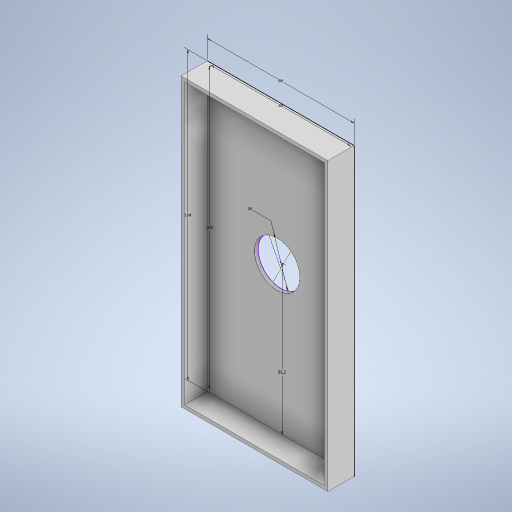
# Autodesk Inventor part: smartphone-holder-aperture26mm
Saved by Autodesk Inventor 2023 (Build 270158000, 158)
## iProperties
Created: 2023-10-02
Part Number: smartphone-holder-aperture26mm
Material: Generic
Document SubType Name: Modeling
Designer: nvladi
Density: 1 g/cm^3
Appearance: Default
Author: nvladi
Autodesk Inventor part; units mm, degrees
ref_plane "YZ Plane" through (0, 0, 0) normal (1, 0, 0) x (0, 1, 0)
ref_plane "XZ Plane" through (0, 0, 0) normal (0, 1, 0) x (-1, 0, 0)
ref_plane "XY Plane" through (0, 0, 0) normal (0, 0, 1) x (1, 0, 0)
sketch "Sketch1" plane through (0, 0, 0) normal (0, 0, 1) x (1, 0, 0)
  line L0 (40, -80) -> (-40, -80)
  line L1 (-40, -80) -> (-40, 80)
  line L2 (-40, 80) -> (40, 80)
  line L3 (40, 80) -> (40, -80)
  line L4 (40, -80) -> (-40, 80) construction
  line L5 (-40, -80) -> (40, 80) construction
  line L6 (42, -82) -> (-42, -82)
  line L7 (-42, -82) -> (-42, 82)
  line L8 (-42, 82) -> (42, 82)
  line L9 (42, 82) -> (42, -82)
  line L10 (42, -82) -> (-42, 82) construction
  line L11 (-42, -82) -> (42, 82) construction
  circle A0 centre (0, 3.2) radius 13
  point P0 (0, 0)
  dimension "d0" = 80
  dimension "d1" = 160
  dimension "d2" = 84
  dimension "d3" = 164
  dimension "d4" = 26
  dimension "d5" = 85.2
  constraints: 24 end point, 4 midpoint, 4 parallel, 2 horizontal, 2 perpendicular, 1 centre point
  measures "d0" distance of L1.end L2.end
  measures "d1" distance of L0.end L1.end
  measures "d2" distance of L7.end L8.end
  measures "d3" distance of L6.end L7.end
  measures "d4" diameter of A0
  measures "d5" distance from line of L6 A0.centre
extrude "Extrusion1" add sketch "Sketch1" along normal blind 2 contours L0 L1 L2 L3
extrude "Extrusion2" add sketch "Sketch1" along normal blind 15 contours L6 L7 L8 L9
body "Solid1"
